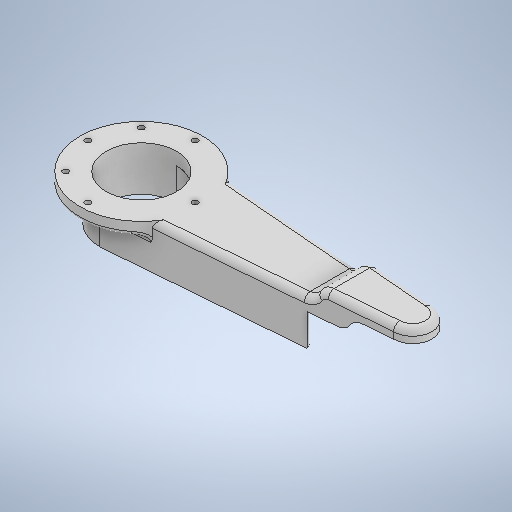
# Autodesk Inventor part: motor3_pulley_case
Saved by Autodesk Inventor 2025 (Build 290162000, 162)
## iProperties
Created: 2025-01-30
Part Number: motor3_pulley_case
Material: Generic
Document SubType Name: Modeling
Designer: danielrachi
Density: 1 g/cm^3
Appearance: Default
Author: danielrachi
Autodesk Inventor part; units mm, degrees
ref_plane "YZ Plane" through (0, 0, 0) normal (1, 0, 0) x (0, 1, 0)
ref_plane "XZ Plane" through (0, 0, 0) normal (0, 1, 0) x (-1, 0, 0)
ref_plane "XY Plane" through (0, 0, 0) normal (0, 0, 1) x (1, 0, 0)
sketch "Sketch1" plane through (0, 0, 0) normal (0, 1, 0) x (-1, 0, 0)
  circle A0 centre (0, 0) radius 32.5
  circle A1 centre (-212.5, 0) radius 15
  line L0 (0, 32.5) -> (-212.5, 15)
  line L1 (0, -32.5) -> (-212.5, -15)
  dimension "d0" = 65
  dimension "d18" = 30
  dimension "d19" = 212.5
  constraints: 4 end point, 4 point on circle, 4 vertical alignment, 2 centre point, 1 coincident, 1 horizontal alignment
  measures "d0" diameter of A0
  measures "d18" diameter of A1
  measures "d19" distance of A1.centre point (0, 0)
extrude "Extrusion4" add sketch "Sketch1" along normal blind 10 contours A0 L1 L0 | A0 L1 A1 L0 | A1
sketch "Sketch4" plane through (0, 10, 0) normal (0, 1, 0) x (1, 0, 0)
  arc A0 (212.5, -15) -> (212.5, 15) centre (212.5, 0) ccw projected
  circle A1 centre (212.5, 0) radius 15
  line L0 (212.5, 15) -> (0, 32.5) projected
  line L1 (157.5, 19.5294) -> (157.5, -19.5294)
  line L2 (0, -32.5) -> (212.5, -15) projected
  point P0 (0, 0)
  point P1 (212.5, 15)
  point P2 (212.5, -15)
  point P3 (212.5, -15)
  point P4 (150, 0)
  point P5 (212.5, 15)
  point P6 (157.5, 0)
  dimension "d61" = 96
  dimension "d22" = 30
  dimension "d28" = 55
  constraints: 2 end point, 2 point on line, 1 centre point, 1 coincident, 1 midpoint, 1 vertical
  measures "d22" diameter of A1
  measures "d28" distance of point (157.5, 0) A1.centre
extrude "Extrusion5" add sketch "Sketch4" along normal blind 10
sketch "Sketch5" plane through (0, 0, 0) normal (0, -1, 0) x (1, 0, 0)
  arc A0 (212.5, -15) -> (212.5, 15) centre (212.5, 0) ccw projected
  circle A1 centre (212.5, 0) radius 15
  point P0 (0, 0)
  point P1 (212.5, 15)
  point P2 (212.5, -15)
  dimension "d25" = 30
  constraints: 1 centre point, 1 coincident
  measures "d25" diameter of A1
extrude "Extrusion6" cut sketch "Sketch5" against normal blind 10
sketch "Sketch6" plane through (0, 10, 0) normal (0, -1, 0) x (1, 0, 0)
  circle A0 centre (212.5, 0) radius 10
  arc A1 (212.5, -15) -> (212.5, 15) centre (212.5, 0) ccw projected
  point P0 (0, 0)
  dimension "d30" = 20
  constraints: 1 centre point, 1 concentric
  measures "d30" diameter of A0
extrude "Extrusion7" cut sketch "Sketch6" against normal blind 6
sketch "Sketch10" plane through (0, 0, 0) normal (0, -1, 0) x (1, 0, 0)
  circle A0 centre (212.5, 0) radius 37.5
  arc A1 (212.5, -15) -> (212.5, 15) centre (212.5, 0) ccw projected
  point P0 (0, 0)
  dimension "d37" = 75
  constraints: 1 centre point, 1 concentric
  measures "d37" diameter of A0
extrude "Extrusion8" cut sketch "Sketch10" against normal up to surface (10 mm away)
fillet "Fillet8" radius 10 4 edges at (175, 0, 0) (175, 10, 0) (157.5, 10, 0) (157.5, 20, 0)
sketch "Sketch14" plane through (0, 0, 0) normal (0, -1, 0) x (1, 0, 0)
  circle A0 centre (0, 0) radius 48
  dimension "d61" = 96
  constraints: 1 centre point, 1 coincident
  measures "d61" diameter of A0
extrude "Extrusion12" add sketch "Sketch14" against normal up to surface (10 mm away)
sketch "Sketch15" plane through (0, 0, 0) normal (0, -1, 0) x (1, 0, 0)
  circle A0 centre (-42, 0) radius 2.25
  circle A1 centre (-29.6985, -29.6985) radius 2.25
  circle A2 centre (0, -42) radius 2.25
  circle A3 centre (29.6985, -29.6985) radius 2.25
  circle A4 centre (42, 0) radius 2.25
  circle A5 centre (29.6985, 29.6985) radius 2.25
  circle A6 centre (0, 42) radius 2.25
  circle A7 centre (-29.6985, 29.6985) radius 2.25
  point P0 (0, 0)
  dimension "d64" = 4.5
  dimension "d65" = 42
  dimension "d68" = 360
  constraints: 8 centre point, 1 horizontal alignment, 17 other
  measures "d64" diameter of A0
  measures "d65" distance of point (0, 0) A0.centre
extrude "Extrusion13" cut sketch "Sketch15" against normal blind 10 contours A0 | A1 | A2 | A4 | A6 | A7
sketch "Sketch16" plane through (0, 0, 0) normal (0, -1, 0) x (1, 0, 0)
  arc A0 (0, 27.5) -> (0, -27.5) centre (0, 0) ccw
  line L0 (0, 0) -> (0, 27.5) construction
  line L1 (0, 0) -> (0, -27.5) construction
  arc A1 (0, 32.5) -> (0, -32.5) centre (0, 0) ccw
  line L2 (0, 0) -> (0, -32.5) construction
  line L3 (0, 0) -> (32.5, 0) construction
  line L4 (0, 0) -> (0, 32.5) construction
  line L5 (171.6156, -18.3669) -> (37.963, -29.3736) projected
  line L6 (0, -32.5) -> (37.963, -29.3736)
  line L7 (37.963, 29.3736) -> (171.6156, 18.3669) projected
  line L8 (0, 32.5) -> (37.963, 29.3736)
  line L9 (0, 27.5) -> (149.4939, 15.1887)
  line L10 (0, -27.5) -> (149.4939, -15.1887)
  line L11 (149.4939, -15.1887) -> (149.9029, -20.1551)
  line L12 (149.4939, 15.1887) -> (149.9029, 20.1551)
  dimension "d72" = 27.5
  dimension "d73" = 180
  dimension "d74" = 32.5
  dimension "d75" = 90
  dimension "d76" = 180
  dimension "d77" = 150
  dimension "d78" = 150
  constraints: 22 end point, 4 point on circle, 3 perpendicular, 2 centre point, 2 coincident, 2 parallel, 2 point on line, 1 horizontal, 1 vertical alignment
  measures "d72" radius of A0
  measures "d73" angle of L0 L1
  measures "d74" radius of A1
  measures "d75" angle of L2 L3
  measures "d76" angle of L2 L4
  measures "d77" distance of L0.end L9.end
  measures "d78" distance of L1.end L10.end
extrude "Extrusion14" add sketch "Sketch16" along normal blind 25
fillet "Fillet9" radius 5 2 edges at (149.4939, -12.5, 15.1887) (149.4939, -12.5, -15.1887)
sketch "Sketch17" plane through (0, -25, 0) normal (0, -1, 0) x (1, 0, 0)
  circle A0 centre (0, -30) radius 1.625
  line L0 (0, -27.5) -> (144.5108, -15.5991) projected
  circle A1 centre (-30, 0) radius 1.625
  circle A2 centre (0, 30) radius 1.625
  line L1 (144.5108, 15.5991) -> (0, 27.5) projected
  line L2 (0, 27.5) -> (144.5108, 15.5991)
  circle A3 centre (49.8313, 25.8962) radius 1.625
  circle A4 centre (99.6626, 21.7925) radius 1.625
  line L3 (0, 0) -> (30.8555, 0)
  circle A5 centre (49.8313, -25.8962) radius 1.625
  circle A6 centre (99.6626, -21.7925) radius 1.625
  dimension "d82" = 3.25
  dimension "d86" = 180
  dimension "d90" = 50
  dimension "d104" = 2.5
  constraints: 7 centre point, 4 end point, 2 symmetric about line, 1 collinear, 1 horizontal, 1 vertical alignment, 12 other
  measures "d82" diameter of A0
  measures "d90" distance of A2.centre A3.centre
  measures "d104" distance of A0.centre L0.start
extrude "Extrusion15" cut sketch "Sketch17" against normal blind 10
fillet "Fillet10" radius 5 3 edges at (-32.5, 0, 0) (18.9815, 0, 30.9368) (18.9815, 0, -30.9368)
fillet "Fillet11" radius 3 3 edges at (36.4211, -1.1931, -31.265) (36.4212, -1.1931, 31.265) (-48, 0, 0)
fillet "Fillet12" radius 5 9 edges at (152.5001, 11.3397, 19.9412) (159.821, 18.6605, 19.3383) (188.6603, 20, 16.9633) (92.7316, 10, 24.8633) (152.5001, 11.3397, -19.9412) (159.821, 18.6605, -19.3383) (188.6603, 20, -16.9633) (92.7316, 10, -24.8633) (227.5, 20, 0)
sketch "Sketch18" plane through (0, 0, 0) normal (0, -1, 0) x (1, 0, 0)
  circle A0 centre (0, 0) radius 27.5
  dimension "d101" = 55
  constraints: 1 centre point, 1 coincident
  measures "d101" diameter of A0
extrude "Extrusion16" cut sketch "Sketch18" against normal through all
equation "\"d0\" = pulley_diameter + thickness"
equation "\"d18\" = bearing_diameter + thickness"
equation "\"d19\" = -0.5 * pulley_diameter + belt_length - 0.5 * bearing_diameter"
equation "\"d20\" = thickness"
equation "\"d61\" = motor_diameter"
equation "\"d22\" = bearing_diameter + thickness"
equation "\"d28\" = pulley_diameter"
equation "\"d25\" = bearing_diameter + thickness"
equation "\"d30\" = bearing_diameter"
equation "\"d31\" = bearing_width"
equation "\"d37\" = pulley_diameter + 2 * thickness"
equation "\"d48\" = thickness"
equation "\"d72\" = 0.5 * pulley_diameter"
equation "\"d74\" = 0.5 * thickness + 0.5 * pulley_diameter"
equation "\"d77\" = wall_length"
equation "\"d78\" = wall_length"
equation "\"d79\" = belt_width"
equation "\"d81\" = 0.5 * thickness"
equation "\"d90\" = 0.333333 * wall_length"
equation "\"d101\" = pulley_diameter"
equation "\"pulley_diameter\" = 55"
equation "\"motor_diameter\" = 96"
equation "\"pulley_width\" = 32"
equation "\"belt_width\" = 25"
equation "\"bearing_to_bearing\" = 64"
equation "\"thickness\" = 10"
equation "\"bearing_diameter\" = 20"
equation "\"bearing_width\" = 6"
equation "\"wall_length\" = 150"
equation "\"belt_length\" = 250"
body "Solid2"
